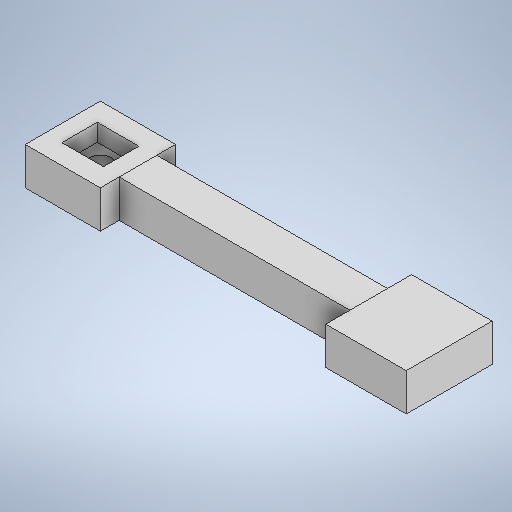
# Autodesk Inventor part: Sensorarm_v2
Saved by Autodesk Inventor 2025 (Build 290162000, 162)
## iProperties
Created: 2026-06-23
Part Number: Sensorarm_v2
Material: Generisch
Document SubType Name: Modeling
Designer: GemmiDad-GBSE
Density: 1 g/cm^3
Appearance: Vorgabe
Author: GemmiDad-GBSE
Autodesk Inventor part; units mm, degrees
ref_plane "YZ Plane" through (0, 0, 0) normal (1, 0, 0) x (0, 1, 0)
sketch "Skizze1" plane through (0, 0, 0) normal (0, 0, 1) x (1, 0, 0)
  line L0 (-14, -14) -> (14, -14)
  line L1 (14, -14) -> (14, 14)
  line L2 (14, 14) -> (-14, 14)
  line L3 (-14, 14) -> (-14, -14)
  constraints: 8 end point, 2 parallel, 1 horizontal, 1 perpendicular
extrude "Extrusion1" add sketch "Skizze1" along normal blind 14
sketch "Skizze2" plane through (0, 0, 0) normal (0, 0, 1) x (1, 0, 0)
  line L0 (14, -7) -> (100, -7)
  line L1 (100, -7) -> (100, 7)
  line L2 (100, 7) -> (14, 7)
  line L3 (14, 7) -> (14, -7)
  constraints: 8 end point, 2 parallel, 1 horizontal, 1 perpendicular
extrude "Extrusion2" add sketch "Skizze2" along normal blind 14 separate body
sketch "Skizze3" plane through (0, 0, 0) normal (0, 0, 1) x (1, 0, 0)
  line L0 (100, -16) -> (130, -16)
  line L1 (130, -16) -> (130, 16)
  line L2 (130, 16) -> (100, 16)
  line L3 (100, 16) -> (100, -16)
  constraints: 8 end point, 2 parallel, 1 horizontal, 1 perpendicular
extrude "Extrusion3" add sketch "Skizze3" along normal blind 14 separate body
sketch "Skizze4" plane through (0, 0, 0) normal (0, 0, 1) x (1, 0, 0)
  circle A0 centre (0, 0) radius 4.25
  constraints: 1 centre point
extrude "Extrusion4" cut sketch "Skizze4" along normal blind 15 bodies 1
ref_plane "Arbeitsebene1" through (0, 0, 14) normal (0, 0, 1) x (1, 0, 0)
sketch "Skizze5" plane through (0, 0, 14) normal (0, 0, 1) x (1, 0, 0)
  line L0 (-7.75, -6.6) -> (7.75, -6.6)
  line L1 (7.75, -6.6) -> (7.75, 6.6)
  line L2 (7.75, 6.6) -> (-7.75, 6.6)
  line L3 (-7.75, 6.6) -> (-7.75, -6.6)
  constraints: 8 end point, 2 parallel, 1 horizontal, 1 perpendicular
extrude "Extrusion5" cut sketch "Skizze5" against normal blind 6.5 bodies 1
sketch "Skizze6" plane through (0, 0, 0) normal (0, 0, 1) x (1, 0, 0)
  line L0 (110.25, -7.75) -> (119.75, -7.75)
  line L1 (119.75, -7.75) -> (119.75, 7.75)
  line L2 (119.75, 7.75) -> (110.25, 7.75)
  line L3 (110.25, 7.75) -> (110.25, -7.75)
  constraints: 8 end point, 2 parallel, 1 horizontal, 1 perpendicular
extrude "Extrusion6" cut sketch "Skizze6" along normal blind 3 bodies 1
sketch "Skizze7" plane through (0, 0, 0) normal (0, 0, 1) x (1, 0, 0)
  circle A0 centre (115, 0) radius 3
  constraints: 1 centre point
extrude "Extrusion7" cut sketch "Skizze7" along normal blind 15 bodies 1
sketch "Skizze8" plane through (0, 0, 0) normal (0, 0, 1) x (1, 0, 0)
  circle A0 centre (105, 0) radius 1.1
  circle A1 centre (125, 0) radius 1.1
  constraints: 2 centre point
extrude "Extrusion8" cut sketch "Skizze8" along normal blind 15 bodies 1
ref_plane "Arbeitsebene2" through (0, 16, 0) normal (0, 1, 0) x (-1, 0, 0)
sketch "Skizze9" plane through (0, 16, 0) normal (0, 1, 0) x (-1, 0, 0)
  line L0 (107.25, 2.25) -> (122.75, 2.25)
  line L1 (122.75, 2.25) -> (122.75, 11.75)
  line L2 (122.75, 11.75) -> (107.25, 11.75)
  line L3 (107.25, 11.75) -> (107.25, 2.25)
  constraints: 8 end point, 2 parallel, 1 horizontal, 1 perpendicular
extrude "Extrusion9" cut sketch "Skizze9" against normal blind 3 bodies 1
sketch "Skizze10" plane through (0, 16, 0) normal (0, 1, 0) x (-1, 0, 0)
  circle A0 centre (115, 7) radius 3
  constraints: 1 centre point
extrude "Extrusion10" cut sketch "Skizze10" along normal mid plane 33 bodies 1
sketch "Skizze11" plane through (0, 16, 0) normal (0, 1, 0) x (-1, 0, 0)
  circle A0 centre (105, 7) radius 1.1
  circle A1 centre (125, 7) radius 1.1
  constraints: 2 centre point
extrude "Extrusion11" cut sketch "Skizze11" along normal mid plane 33 bodies 1
